Autodesk Fusion 360 part; units mm, degrees
note: some values were not read from the file. Chosen so that the rebuilt part matches the saved one: that a step has no effect; which bodies a step acts on.
(part 3 of 3)
  spline S44 degree 5 poles (74.3724, 79.3275) (74.4983, 79.3959) (74.7869, 79.4495) (75.3331, 79.2791) (76.2877, 78.5722) (77.8111, 77.037) (79.5761, 75.0532) (81.4574, 72.8394) (83.2976, 70.5938) (84.9099, 68.4508) (86.1037, 66.4908) (86.7156, 64.7591) (86.6405, 63.2818) (85.8582, 62.0812) (84.4763, 61.195) (82.7145, 60.6783) (80.8322, 60.5883) (79.0753, 60.9749) (77.61, 61.8677) (76.478, 63.2653) (75.644, 65.1321) (75.0293, 67.3929) (74.5505, 69.9277) (74.1551, 72.5664) (73.8599, 75.0817) (73.7271, 77.2261) (73.8174, 78.4613) (74.0317, 79.0393) (74.2465, 79.2592) (74.3724, 79.3275) knots 0 0 0 0 0 0 0.04 0.08 0.12 0.16 0.2 0.24 0.28 0.32 0.36 0.4 0.44 0.48 0.52 0.56 0.6 0.64 0.68 0.72 0.76 0.8 0.84 0.88 0.92 0.96 1 1 1 1 1 1
  spline S45 degree 5 poles (77.0951, 83.174) (77.1541, 83.3575) (77.3433, 83.6926) (77.8394, 84.1026) (78.903, 84.488) (80.7683, 84.7946) (82.9906, 85.0245) (85.3767, 85.253) (87.752, 85.4996) (89.9857, 85.7085) (91.9839, 85.7812) (93.6881, 85.6017) (95.0712, 85.0647) (96.1349, 84.1011) (96.9078, 82.7096) (97.4352, 80.948) (97.7677, 78.9142) (97.9496, 76.7301) (98.009, 74.5261) (97.9427, 72.423) (97.7237, 70.5254) (97.3172, 68.9202) (96.6946, 67.6735) (95.8467, 66.8283) (94.8022, 66.4002) (93.6138, 66.3826) (92.3321, 66.7544) (90.9793, 67.4888) (89.5402, 68.5566) (87.9881, 69.9216) (86.3007, 71.5383) (84.4818, 73.348) (82.5776, 75.2763) (80.7031, 77.2274) (79.0254, 79.0936) (77.7281, 80.7716) (77.1314, 81.8953) (76.9889, 82.5917) (77.036, 82.9905) (77.0951, 83.174) knots 0 0 0 0 0 0 0.028571 0.057143 0.085714 0.114286 0.142857 0.171429 0.2 0.228571 0.257143 0.285714 0.314286 0.342857 0.371429 0.4 0.428571 0.457143 0.485714 0.514286 0.542857 0.571429 0.6 0.628571 0.657143 0.685714 0.714286 0.742857 0.771429 0.8 0.828571 0.857143 0.885714 0.914286 0.942857 0.971429 1 1 1 1 1 1
  spline S46 degree 5 poles (23.5329, 74.9821) (23.5506, 75.3613) (23.5819, 76.1216) (23.6138, 77.2541) (23.6391, 78.6838) (23.7372, 80.1667) (24.0204, 81.1917) (24.5917, 81.6461) (25.4957, 81.4872) (26.689, 80.7599) (28.0697, 79.5668) (29.4963, 78.0467) (30.811, 76.3495) (31.8599, 74.615) (32.516, 72.9464) (32.6896, 71.4159) (32.3371, 70.0736) (31.4726, 68.956) (30.1766, 68.0934) (28.6123, 67.5191) (26.9896, 67.2661) (25.5219, 67.3622) (24.3839, 67.8252) (23.6704, 68.6579) (23.3515, 69.8425) (23.3177, 71.3389) (23.4047, 72.7328) (23.4753, 73.8467) (23.5151, 74.6029) (23.5329, 74.9821) knots 0 0 0 0 0 0 0.04 0.08 0.12 0.16 0.2 0.24 0.28 0.32 0.36 0.4 0.44 0.48 0.52 0.56 0.6 0.64 0.68 0.72 0.76 0.8 0.84 0.88 0.92 0.96 1 1 1 1 1 1
  spline S47 degree 5 poles (9.5628, 80.1303) (10.0078, 80.438) (10.8978, 81.0432) (12.2172, 81.9077) (13.8963, 82.912) (15.791, 83.751) (17.444, 84.0225) (18.8338, 83.6284) (19.9372, 82.5571) (20.7119, 80.9213) (21.1057, 78.9157) (21.0668, 76.7718) (20.5534, 74.7171) (19.5452, 72.927) (18.0513, 71.4998) (16.1143, 70.4796) (13.8156, 69.868) (11.2803, 69.639) (8.6837, 69.7524) (6.2559, 70.167) (4.2415, 70.8422) (2.862, 71.74) (2.2782, 72.8266) (2.5481, 74.0751) (3.5957, 75.4655) (5.2576, 76.9731) (6.9085, 78.2411) (8.2278, 79.197) (9.1178, 79.8226) (9.5628, 80.1303) knots 0 0 0 0 0 0 0.04 0.08 0.12 0.16 0.2 0.24 0.28 0.32 0.36 0.4 0.44 0.48 0.52 0.56 0.6 0.64 0.68 0.72 0.76 0.8 0.84 0.88 0.92 0.96 1 1 1 1 1 1
  spline S48 degree 5 poles (31.4167, 84.1146) (31.568, 84.2032) (31.9062, 84.3291) (32.5145, 84.3598) (33.4918, 84.0829) (34.8685, 83.2545) (36.2642, 82.03) (37.5479, 80.5204) (38.6121, 78.8491) (39.3937, 77.1384) (39.8871, 75.4986) (40.1212, 74.026) (40.1431, 72.7987) (39.9983, 71.8738) (39.7153, 71.2837) (39.2817, 71.0303) (38.6631, 71.096) (37.8398, 71.4623) (36.8318, 72.1233) (35.6887, 73.0736) (34.4821, 74.3001) (33.2977, 75.7712) (32.2281, 77.4287) (31.3647, 79.1737) (30.7903, 80.871) (30.5709, 82.3727) (30.7119, 83.3036) (30.9987, 83.7972) (31.2655, 84.026) (31.4167, 84.1146) knots 0 0 0 0 0 0 0.04 0.08 0.12 0.16 0.2 0.24 0.28 0.32 0.36 0.4 0.44 0.48 0.52 0.56 0.6 0.64 0.68 0.72 0.76 0.8 0.84 0.88 0.92 0.96 1 1 1 1 1 1
  spline S49 degree 5 poles (54.7523, 85.1815) (54.9089, 85.6313) (55.2214, 86.5284) (55.6833, 87.8587) (56.2744, 89.5712) (56.9682, 91.5414) (57.6297, 93.2825) (58.2832, 94.7476) (58.9577, 95.9027) (59.6812, 96.7284) (60.4744, 97.222) (61.345, 97.3987) (62.2897, 97.2858) (63.2974, 96.9181) (64.3513, 96.3314) (65.4308, 95.5593) (66.5117, 94.6355) (67.5671, 93.5945) (68.5673, 92.4735) (69.4806, 91.313) (70.274, 90.1585) (70.9188, 89.0535) (71.3968, 88.0334) (71.7059, 87.1193) (71.8667, 86.3107) (71.9263, 85.581) (71.9276, 84.891) (71.8846, 84.201) (71.7503, 83.4842) (71.4519, 82.726) (70.9261, 81.9219) (70.1618, 81.0763) (69.1927, 80.2) (68.0763, 79.3078) (66.8766, 78.4153) (65.6467, 77.5368) (64.407, 76.6822) (63.1497, 75.8581) (61.8541, 75.0729) (60.4987, 74.34) (59.0753, 73.6817) (57.6007, 73.1329) (56.1334, 72.7461) (54.7634, 72.5848) (53.5899, 72.7124) (52.7033, 73.1813) (52.166, 74.0233) (51.9906, 75.2375) (52.1479, 76.7941) (52.5801, 78.6408) (53.2118, 80.7091) (53.8118, 82.4775) (54.2815, 83.8298) (54.5956, 84.7318) (54.7523, 85.1815) knots 0 0 0 0 0 0 0.02 0.04 0.06 0.08 0.1 0.12 0.14 0.16 0.18 0.2 0.22 0.24 0.26 0.28 0.3 0.32 0.34 0.36 0.38 0.4 0.42 0.44 0.46 0.48 0.5 0.52 0.54 0.56 0.58 0.6 0.62 0.64 0.66 0.68 0.7 0.72 0.74 0.76 0.78 0.8 0.82 0.84 0.86 0.88 0.9 0.92 0.94 0.96 0.98 1 1 1 1 1 1
  spline S50 degree 5 poles (37.4267, 87.4813) (37.5322, 87.7415) (37.7986, 88.2561) (38.3653, 89.0064) (39.436, 89.9413) (41.1771, 90.9151) (43.1513, 91.5963) (45.1688, 91.8918) (47.0458, 91.729) (48.6343, 91.0748) (49.8396, 89.945) (50.6107, 88.3928) (50.9371, 86.5011) (50.8431, 84.3746) (50.3841, 82.1317) (49.6414, 79.8969) (48.7108, 77.7943) (47.6915, 75.9412) (46.6752, 74.4421) (45.7342, 73.3814) (44.9115, 72.8176) (44.2065, 72.7752) (43.5839, 73.2418) (42.9893, 74.1642) (42.3618, 75.4465) (41.6489, 76.9706) (40.8207, 78.614) (39.8845, 80.2689) (38.8997, 81.8603) (37.9923, 83.3654) (37.321, 84.7929) (37.0993, 85.8901) (37.166, 86.6945) (37.3213, 87.221) (37.4267, 87.4813) knots 0 0 0 0 0 0 0.033333 0.066667 0.1 0.133333 0.166667 0.2 0.233333 0.266667 0.3 0.333333 0.366667 0.4 0.433333 0.466667 0.5 0.533333 0.566667 0.6 0.633333 0.666667 0.7 0.733333 0.766667 0.8 0.833333 0.866667 0.9 0.933333 0.966667 1 1 1 1 1 1
  spline S51 degree 5 poles (5.382, 90.2931) (5.6237, 90.4332) (6.1142, 90.6822) (6.8649, 90.9621) (7.8762, 91.162) (9.1269, 91.2039) (10.3449, 91.1387) (11.5159, 91.0587) (12.6242, 91.0235) (13.6452, 91.0266) (14.5458, 91.0081) (15.2877, 90.8878) (15.8307, 90.5893) (16.1349, 90.0738) (16.1654, 89.3412) (15.897, 88.4192) (15.3196, 87.3543) (14.4398, 86.2062) (13.2807, 85.0434) (11.8818, 83.9396) (10.2998, 82.9689) (8.6081, 82.2022) (6.8988, 81.7024) (5.2797, 81.5207) (3.8615, 81.6901) (2.7457, 82.2207) (2.012, 83.0931) (1.7067, 84.2535) (1.8276, 85.6046) (2.3305, 87.0192) (3.1445, 88.3623) (3.9766, 89.281) (4.6639, 89.8415) (5.1403, 90.1529) (5.382, 90.2931) knots 0 0 0 0 0 0 0.033333 0.066667 0.1 0.133333 0.166667 0.2 0.233333 0.266667 0.3 0.333333 0.366667 0.4 0.433333 0.466667 0.5 0.533333 0.566667 0.6 0.633333 0.666667 0.7 0.733333 0.766667 0.8 0.833333 0.866667 0.9 0.933333 0.966667 1 1 1 1 1 1
  spline S52 degree 5 poles (21.4048, 94.5619) (21.5679, 94.772) (21.9013, 95.1893) (22.4187, 95.801) (23.1284, 96.5615) (24.0224, 97.3465) (24.9072, 97.8944) (25.7765, 98.1473) (26.6333, 98.0712) (27.4904, 97.6698) (28.3647, 96.9813) (29.2697, 96.0673) (30.208, 95.0034) (31.1636, 93.87) (32.0948, 92.7426) (32.9258, 91.6825) (33.5649, 90.7343) (33.9225, 89.9248) (33.9309, 89.2602) (33.5609, 88.725) (32.8445, 88.2787) (31.8586, 87.8676) (30.7045, 87.4396) (29.4881, 86.9582) (28.301, 86.4154) (27.1985, 85.8486) (26.2044, 85.3248) (25.3185, 84.9219) (24.5237, 84.7097) (23.7926, 84.733) (23.0941, 84.9889) (22.4016, 85.4352) (21.7009, 86.0135) (20.9973, 86.666) (20.3269, 87.3585) (19.7491, 88.0816) (19.3285, 88.8403) (19.1221, 89.6476) (19.1616, 90.5163) (19.4431, 91.452) (19.9385, 92.4516) (20.4704, 93.2905) (20.9229, 93.9285) (21.2418, 94.3517) (21.4048, 94.5619) knots 0 0 0 0 0 0 0.025 0.05 0.075 0.1 0.125 0.15 0.175 0.2 0.225 0.25 0.275 0.3 0.325 0.35 0.375 0.4 0.425 0.45 0.475 0.5 0.525 0.55 0.575 0.6 0.625 0.65 0.675 0.7 0.725 0.75 0.775 0.8 0.825 0.85 0.875 0.9 0.925 0.95 0.975 1 1 1 1 1 1
  spline S53 degree 5 poles (9.5224, 94.651) (9.5534, 94.7589) (9.6487, 94.9598) (9.8892, 95.2082) (10.3785, 95.4069) (11.153, 95.4008) (11.9467, 95.1388) (12.6172, 94.6532) (13.0497, 94.0121) (13.1852, 93.3236) (13.0137, 92.7131) (12.5668, 92.2979) (11.9115, 92.1649) (11.1481, 92.3397) (10.4016, 92.7772) (9.7994, 93.39) (9.5221, 93.9308) (9.4627, 94.3126) (9.4914, 94.5432) (9.5224, 94.651) knots 0 0 0 0 0 0 0.066667 0.133333 0.2 0.266667 0.333333 0.4 0.466667 0.533333 0.6 0.666667 0.733333 0.8 0.866667 0.933333 1 1 1 1 1 1
  spline S54 degree 5 poles (8.0856, 98.2896) (8.1791, 98.1795) (8.3474, 97.9487) (8.5418, 97.5719) (8.6816, 97.0145) (8.659, 96.2364) (8.4474, 95.3929) (8.0597, 94.5131) (7.5099, 93.6507) (6.8141, 92.8792) (5.9943, 92.2769) (5.0818, 91.9148) (4.1195, 91.8447) (3.1675, 92.0837) (2.3013, 92.6085) (1.5999, 93.3682) (1.1346, 94.2926) (0.958, 95.3019) (1.092, 96.3166) (1.5188, 97.2655) (2.1926, 98.0875) (3.0485, 98.7341) (4.0117, 99.172) (5.0065, 99.3857) (5.9664, 99.3812) (6.8355, 99.1807) (7.4222, 98.8881) (7.7861, 98.6088) (7.992, 98.3996) (8.0856, 98.2896) knots 0 0 0 0 0 0 0.04 0.08 0.12 0.16 0.2 0.24 0.28 0.32 0.36 0.4 0.44 0.48 0.52 0.56 0.6 0.64 0.68 0.72 0.76 0.8 0.84 0.88 0.92 0.96 1 1 1 1 1 1
  spline S55 degree 5 poles (82.4719, 94.0234) (82.859, 94.3096) (83.6253, 94.8875) (84.7368, 95.7586) (86.1004, 96.8667) (87.5579, 97.983) (88.7575, 98.6588) (89.7084, 98.7674) (90.4232, 98.2594) (90.8971, 97.2091) (91.1082, 95.7864) (91.0252, 94.1987) (90.6131, 92.6476) (89.8388, 91.2697) (88.6811, 90.1325) (87.1436, 89.2567) (85.2674, 88.6302) (83.1422, 88.2242) (80.9253, 88.0099) (78.8371, 87.9691) (77.1147, 88.0917) (75.9734, 88.3761) (75.5667, 88.8284) (75.9406, 89.4629) (77.008, 90.2991) (78.5997, 91.3479) (80.1208, 92.3487) (81.3028, 93.1703) (82.0848, 93.7372) (82.4719, 94.0234) knots 0 0 0 0 0 0 0.04 0.08 0.12 0.16 0.2 0.24 0.28 0.32 0.36 0.4 0.44 0.48 0.52 0.56 0.6 0.64 0.68 0.72 0.76 0.8 0.84 0.88 0.92 0.96 1 1 1 1 1 1
  spline S56 degree 5 poles (19.209, 95.7159) (19.1796, 95.5166) (19.0882, 95.1151) (18.8602, 94.5132) (18.4081, 93.7521) (17.7039, 92.9797) (16.9654, 92.4844) (16.2724, 92.3341) (15.6515, 92.5431) (15.0624, 93.0596) (14.4359, 93.7932) (13.7076, 94.6375) (12.848, 95.492) (11.9054, 96.2892) (11.0023, 97) (10.2916, 97.6178) (9.9218, 98.1487) (10.003, 98.6006) (10.5624, 98.9703) (11.5425, 99.2415) (12.8314, 99.391) (14.2833, 99.3933) (15.7424, 99.2248) (17.0656, 98.8694) (18.1422, 98.3225) (18.8938, 97.5941) (19.2013, 96.8882) (19.265, 96.3112) (19.2385, 95.9153) (19.209, 95.7159) knots 0 0 0 0 0 0 0.04 0.08 0.12 0.16 0.2 0.24 0.28 0.32 0.36 0.4 0.44 0.48 0.52 0.56 0.6 0.64 0.68 0.72 0.76 0.8 0.84 0.88 0.92 0.96 1 1 1 1 1 1
  spline S57 degree 5 poles (80.9043, 94.7369) (80.6785, 94.495) (80.144, 94.0377) (79.1107, 93.4506) (77.3787, 92.9273) (75.0082, 92.7836) (72.859, 93.1607) (71.3246, 94.0046) (70.6988, 95.2012) (71.0831, 96.5706) (72.3635, 97.8822) (74.2912, 98.9009) (76.5307, 99.4258) (78.7153, 99.3313) (80.4982, 98.6173) (81.6001, 97.4387) (81.7845, 96.3143) (81.4985, 95.4891) (81.13, 94.9788) (80.9043, 94.7369) knots 0 0 0 0 0 0 0.066667 0.133333 0.2 0.266667 0.333333 0.4 0.466667 0.533333 0.6 0.666667 0.733333 0.8 0.866667 0.933333 1 1 1 1 1 1
  spline S58 degree 5 poles (96.536, 88.1146) (96.3472, 88.1201) (95.9663, 88.1839) (95.3941, 88.4383) (94.6663, 89.0805) (93.9028, 90.3021) (93.3618, 91.8198) (93.1001, 93.4865) (93.1475, 95.1443) (93.497, 96.6362) (94.1096, 97.8182) (94.9228, 98.5712) (95.8579, 98.814) (96.8262, 98.5163) (97.7359, 97.7136) (98.4994, 96.4919) (99.0404, 94.9743) (99.3021, 93.3075) (99.2547, 91.6497) (98.9052, 90.1578) (98.2927, 88.9758) (97.642, 88.3734) (97.0993, 88.1513) (96.7249, 88.1092) (96.536, 88.1146) knots 0 0 0 0 0 0 0.05 0.1 0.15 0.2 0.25 0.3 0.35 0.4 0.45 0.5 0.55 0.6 0.65 0.7 0.75 0.8 0.85 0.9 0.95 1 1 1 1 1 1
  spline S59 degree 5 poles (56.0235, 99.0275) (56.0646, 98.8768) (56.0421, 98.5562) (55.6924, 98.0243) (54.6123, 97.247) (52.3863, 96.2594) (49.5085, 95.3555) (46.2558, 94.627) (42.9358, 94.1451) (39.8641, 93.9518) (37.3386, 94.0618) (35.6135, 94.4647) (34.8722, 95.125) (35.1993, 95.9831) (36.5494, 96.9547) (38.7754, 97.9424) (41.6532, 98.8462) (44.9059, 99.5748) (48.2259, 100.0566) (51.2976, 100.25) (53.8231, 100.1399) (55.2032, 99.8176) (55.7955, 99.46) (55.9824, 99.1781) (56.0235, 99.0275) knots 0 0 0 0 0 0 0.05 0.1 0.15 0.2 0.25 0.3 0.35 0.4 0.45 0.5 0.55 0.6 0.65 0.7 0.75 0.8 0.85 0.9 0.95 1 1 1 1 1 1
  line L0 (0, 0) -> (100, 0)
  line L1 (100, 0) -> (100, 100)
  line L2 (100, 100) -> (0, 100)
  line L3 (0, 100) -> (0, 0)
  point P0 (30.9151, 1.2041)
  point P1 (17.332, 0.3633)
  point P2 (3.435, 2.4291)
  point P3 (76.9257, 7.1373)
  point P4 (79.4091, 4.1244)
  point P5 (75.0431, 0.793)
  point P6 (93.1072, 7.659)
  point P7 (97.9381, 2.5312)
  point P8 (90.2734, 0.9991)
  point P9 (82.1503, 4.3305)
  point P10 (12.4278, 13.2269)
  point P11 (25.0087, 13.3144)
  point P12 (29.5981, 7.528)
  point P13 (16.5849, 4.8588)
  point P14 (3.0018, 8.5301)
  point P15 (58.8273, 13.8811)
  point P16 (64.3481, 12.9504)
  point P17 (71.1952, 9.8471)
  point P18 (70.2267, 4.7078)
  point P19 (62.9347, 1.6949)
  point P20 (42.9422, 16.1994)
  point P21 (48.0981, 16.2741)
  point P22 (51.6654, 15.1953)
  point P23 (54.2776, 8.1239)
  point P24 (45.2159, 2.0539)
  point P25 (36.239, 2.8947)
  point P26 (35.3552, 7.6296)
  point P27 (79.2326, 23.9138)
  point P28 (82.3409, 25.3969)
  point P29 (83.364, 23.2183)
  point P30 (85.3606, 17.4183)
  point P31 (83.0446, 12.0005)
  point P32 (77.7274, 9.8856)
  point P33 (74.3299, 11.6936)
  point P34 (67.8008, 22.6526)
  point P35 (71.7976, 18.3516)
  point P36 (64.7382, 15.0231)
  point P37 (98.6703, 13.7283)
  point P38 (93.8393, 9.7271)
  point P39 (88.0323, 16.9443)
  point P40 (19.1097, 27.0318)
  point P41 (20.7173, 21.9097)
  point P42 (12.5966, 15.5309)
  point P43 (91.9879, 28.8677)
  point P44 (98.123, 26.1144)
  point P45 (92.316, 23.1212)
  point P46 (85.4885, 24.9201)
  point P47 (41.7985, 29.6032)
  point P48 (46.3092, 25.8185)
  point P49 (42.6257, 19.0064)
  point P50 (55.5269, 27.7084)
  point P51 (59.8676, 24.4417)
  point P52 (58.7122, 19.8955)
  point P53 (57.1882, 16.5252)
  point P54 (54.1312, 17.4803)
  point P55 (48.4072, 32.1233)
  point P56 (49.7463, 25.2468)
  point P57 (48.9957, 19.6886)
  point P58 (47.5232, 26.4259)
  point P59 (32.7535, 28.6644)
  point P60 (35.6808, 22.3955)
  point P61 (33.8132, 16.1968)
  point P62 (28.015, 15.8274)
  point P63 (23.5548, 22.1187)
  point P64 (13.6106, 30.6833)
  point P65 (9.0949, 21.1286)
  point P66 (1.7089, 13.8913)
  point P67 (1.2766, 21.4518)
  point P68 (66.6019, 34.7321)
  point P69 (74.3213, 31.7483)
  point P70 (76.9632, 26.1576)
  point P71 (68.2761, 24.6702)
  point P72 (62.3721, 25.8879)
  point P73 (89.3754, 35.7974)
  point P74 (95.085, 36.1515)
  point P75 (98.4764, 32.2173)
  point P76 (92.3413, 30.2827)
  point P77 (20.3331, 40.8013)
  point P78 (26.2881, 43.5376)
  point P79 (27.4212, 38.1219)
  point P80 (24.7077, 31.5355)
  point P81 (20.2291, 30.0193)
  point P82 (16.6241, 33.1953)
  point P83 (50.7404, 37.9025)
  point P84 (55.6101, 39.0182)
  point P85 (59.8065, 36.3104)
  point P86 (60.4517, 31.5446)
  point P87 (55.1434, 30.3401)
  point P88 (49.5918, 33.6255)
  point P89 (44.742, 36.2783)
  point P90 (45.2432, 35.3168)
  point P91 (45.0731, 34.8129)
  point P92 (41.3453, 31.7986)
  point P93 (34.7346, 31.2555)
  point P94 (31.1203, 37.9345)
  point P95 (95.2204, 42.814)
  point P96 (97.6652, 43.1087)
  point P97 (99.2572, 39.3773)
  point P98 (95.8658, 37.6491)
  point P99 (76.3229, 39.4169)
  point P100 (83.0215, 36.6467)
  point P101 (84.0381, 32.1219)
  point P102 (82.9202, 29.5869)
  point P103 (82.2252, 28.6324)
  point P104 (76.4751, 32.74)
  point P105 (74.791, 46.0609)
  point P106 (80.0383, 43.7918)
  point P107 (75.4657, 41.3846)
  point P108 (66.3266, 47.9991)
  point P109 (67.5825, 47.0286)
  point P110 (68.3866, 43.3947)
  point P111 (68.2079, 39.7539)
  point P112 (66.0665, 37.4325)
  point P113 (62.1592, 37.8254)
  point P114 (59.4193, 46.1402)
  point P115 (61.4366, 43.7624)
  point P116 (56.3455, 40.7351)
  point P117 (10.9687, 40.3673)
  point P118 (11.7064, 37.1737)
  point P119 (6.3949, 34.5053)
  point P120 (1.447, 42.5741)
  point P121 (33.0606, 47.996)
  point P122 (39.2214, 48.299)
  point P123 (41.932, 43.0299)
  point P124 (36.3019, 41.6162)
  point P125 (28.9259, 45.388)
  point P126 (88.5517, 46.9065)
  point P127 (91.4302, 41.3322)
  point P128 (88.1654, 37.685)
  point P129 (84.4051, 38.4155)
  point P130 (82.279, 43.5929)
  point P131 (50.7251, 48.3232)
  point P132 (51.9265, 46.3524)
  point P133 (52.5601, 43.1585)
  point P134 (49.7077, 39.6649)
  point P135 (46.5612, 37.955)
  point P136 (44.8125, 42.6687)
  point P137 (20.4577, 49.3656)
  point P138 (24.9249, 47.6251)
  point P139 (25.4247, 46.5616)
  point P140 (20.0004, 42.7146)
  point P141 (13.4791, 41.4291)
  point P142 (11.7886, 48.2714)
  point P143 (5.5201, 50.0785)
  point P144 (1.3098, 55.8487)
  point P145 (98.0739, 63.021)
  point P146 (99.6091, 54.6607)
  point P147 (98.0171, 45.8391)
  point P148 (88.537, 59.8039)
  point P149 (93.0839, 62.1868)
  point P150 (95.0801, 54.1964)
  point P151 (94.1706, 45.5413)
  point P152 (89.4926, 49.2438)
  point P153 (55.6258, 53.8151)
  point P154 (61.5453, 54.4807)
  point P155 (65.3208, 51.4549)
  point P156 (64.9709, 49.672)
  point P157 (59.6809, 47.6112)
  point P158 (53.9562, 47.7778)
  point P159 (41.3299, 52.3024)
  point P160 (45.8478, 51.2018)
  point P161 (45.7311, 48.9199)
  point P162 (40.8317, 49.3215)
  point P163 (72.5346, 57.4638)
  point P164 (78.5076, 57.7982)
  point P165 (82.5556, 55.2631)
  point P166 (80.802, 50.5211)
  point P167 (74.673, 47.9463)
  point P168 (69.2964, 49.173)
  point P169 (68.3903, 51.9264)
  point P170 (49.4776, 53.5243)
  point P171 (51.1601, 50.9792)
  point P172 (50.681, 49.9921)
  point P173 (47.074, 51.4872)
  point P174 (22.0448, 65.1658)
  point P175 (23.3689, 57.95)
  point P176 (19.4653, 52.2123)
  point P177 (9.2336, 55.6334)
  point P178 (2.965, 62.6792)
  point P179 (41.1894, 68.8999)
  point P180 (43.3974, 69.3887)
  point P181 (45.518, 63.2367)
  point P182 (44.4868, 56.1182)
  point P183 (41.3274, 54.6373)
  point P184 (38.1679, 67.3689)
  point P185 (38.3139, 60.355)
  point P186 (37.8742, 52.5955)
  point P187 (32.8315, 50.4414)
  point P188 (27.6663, 50.0077)
  point P189 (27.1027, 57.4858)
  point P190 (49.9664, 68.9326)
  point P191 (54.2481, 63.271)
  point P192 (53.8444, 56.2239)
  point P193 (49.77, 55.6895)
  point P194 (47.039, 63.3524)
  point P195 (64.9796, 64.142)
  point P196 (66.9912, 56.8659)
  point P197 (62.0587, 56.7109)
  point P198 (56.5429, 63.0924)
  point P199 (72.6248, 69.6907)
  point P200 (71.5439, 60.3276)
  point P201 (66.5451, 65.2472)
  point P202 (81.7585, 72.4555)
  point P203 (86.1828, 62.7423)
  point P204 (79.4531, 60.9896)
  point P205 (74.5609, 70.0182)
  point P206 (84.8973, 85.2095)
  point P207 (95.247, 84.7874)
  point P208 (97.9512, 76.0265)
  point P209 (96.416, 67.4872)
  point P210 (92.8278, 66.6561)
  point P211 (83.8566, 73.9863)
  point P212 (24.5212, 81.4472)
  point P213 (30.9132, 76.0897)
  point P214 (31.1895, 68.8655)
  point P215 (24.4646, 67.9348)
  point P216 (18.8032, 83.4356)
  point P217 (20.6672, 75.4683)
  point P218 (11.4267, 69.7292)
  point P219 (2.5192, 72.7121)
  point P220 (38.338, 79.1992)
  point P221 (39.8995, 71.7623)
  point P222 (38.7148, 71.1433)
  point P223 (32.7741, 76.631)
  point P224 (59.6777, 96.6273)
  point P225 (62.9405, 97.02)
  point P226 (68.5076, 92.5088)
  point P227 (71.6437, 87.2352)
  point P228 (71.9143, 84.8418)
  point P229 (71.2896, 82.5262)
  point P230 (66.4794, 78.1365)
  point P231 (58.6329, 73.5367)
  point P232 (52.6801, 73.3853)
  point P233 (46.403, 91.7137)
  point P234 (50.772, 84.5139)
  point P235 (45.5652, 73.3334)
  point P236 (43.6518, 73.2894)
  point P237 (39.8823, 80.2375)
  point P238 (11.8414, 91.0542)
  point P239 (15.4424, 90.761)
  point P240 (16.0266, 88.9797)
  point P241 (9.0342, 82.4374)
  point P242 (1.9906, 83.4575)
  point P243 (26.0728, 98.0761)
  point P244 (31.1916, 93.8301)
  point P245 (33.8062, 89.2051)
  point P246 (29.3405, 86.8766)
  point P247 (24.3059, 84.7505)
  point P248 (21.4536, 86.2526)
  point P249 (19.2056, 89.4896)
  point P250 (12.5904, 94.5811)
  point P251 (12.1339, 92.2539)
  point P252 (8.2827, 95.0686)
  point P253 (4.4348, 91.9103)
  point P254 (1.0434, 95.1312)
  point P255 (4.2377, 99.1833)
  point P256 (89.8748, 98.5346)
  point P257 (90.8349, 93.6655)
  point P258 (83.8592, 88.3919)
  point P259 (75.7864, 88.7498)
  point P260 (16.4255, 92.425)
  point P261 (13.281, 95.0455)
  point P262 (10.0159, 98.3364)
  point P263 (15.4109, 99.2301)
  point P264 (71.0828, 94.7369)
  point P265 (78.1955, 99.2481)
  point P266 (93.162, 93.8103)
  point P267 (95.8662, 98.6794)
  point P268 (99.2402, 92.9838)
  point P269 (46.7292, 94.7815)
  point P270 (35.1382, 95.1742)
  point P271 (44.4325, 99.4202)
extrude "Extrude13" cut sketch "Voronoi - Sketch2" against normal blind 100 contours S1 | S3 | S4 | S9 | S10 | S11 | S13 | S18 | S22 | S28 | S29 | S31 | S34 | S36 | S38 | S39 | S41 | S42 | S46 | S47 | S48 | S49 | S52 | S55 | S57 bodies 2
move_body "Move2" bodies 2 to x (1, 0, 0) y (0, 1, 0) z (0, 0, 1) at (-30, 0, 0)
